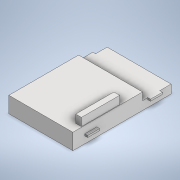
# Autodesk Inventor part: Screen_Model
Saved by Autodesk Inventor 2021 (Build 250183000, 183)
## iProperties
Created: 2020-07-08
Part Number: Screen_Model
Material: Generic
Document SubType Name: Modeling
Designer: ameli
Density: 1 g/cm^3
Appearance: Default
Author: ameli
Autodesk Inventor part; units mm, degrees
ref_plane "YZ Plane" through (0, 0, 0) normal (1, 0, 0) x (0, 1, 0)
ref_plane "XZ Plane" through (0, 0, 0) normal (0, 1, 0) x (-1, 0, 0)
ref_plane "XY Plane" through (0, 0, 0) normal (0, 0, 1) x (1, 0, 0)
sketch "Sketch1" plane through (0, 0, 0) normal (0, 1, 0) x (-1, 0, 0)
  line L0 (28, 43) -> (-28, 43)
  line L1 (-28, 43) -> (-28, -43)
  line L2 (-28, -43) -> (28, -43)
  line L3 (28, -43) -> (28, 43)
  point P0 (0, 0)
  dimension "d0" = 56
  dimension "d1" = 86
  dimension "d4" = 28
  dimension "d5" = 43
  constraints: 8 end point, 2 parallel, 1 horizontal, 1 perpendicular
  measures "d0" distance of L1.end L2.end
  measures "d1" distance of L2.end L0.start
  measures "d4" distance from line of point (0, 0) L3
  measures "d5" distance from line of point (0, 0) L2
extrude "Extrusion1" add sketch "Sketch1" along normal blind 7.5
sketch "Sketch3" plane through (0, 7.5, 0) normal (0, 1, 0) x (1, 0, 0)
  line L0 (22.5, -35) -> (27.5, -35)
  line L1 (27.5, -35) -> (27.5, -1.5)
  line L2 (27.5, -1.5) -> (22.5, -1.5)
  line L3 (22.5, -1.5) -> (22.5, -35)
  line L4 (-28, -43) -> (28, -43) projected
  line L5 (28, -43) -> (28, 43) projected
  point P0 (0, 0)
  dimension "d6" = 33.5
  dimension "d7" = 5
  dimension "d8" = 8
  dimension "d9" = 0.5
  constraints: 8 end point, 2 parallel, 1 horizontal, 1 perpendicular
  measures "d6" distance of L2.end L0.start
  measures "d7" distance of L1.end L2.end
  measures "d8" distance between parallel lines of L4 L0
  measures "d9" distance between parallel lines of L5 L1
extrude "Extrusion2" add sketch "Sketch3" along normal blind 13.5
sketch "Sketch4" plane through (0, 7.5, 0) normal (0, 1, 0) x (1, 0, 0)
  line L0 (-28, 43) -> (-28, -43) projected
  line L1 (-30.4, -32.5) -> (-28, -32.5)
  line L2 (-28, -32.5) -> (-28, -22)
  line L3 (-28, -22) -> (-30.4, -22)
  line L4 (-30.4, -22) -> (-30.4, -32.5)
  line L5 (-30.4, 22.5) -> (-28, 22.5)
  line L6 (-28, 22.5) -> (-28, 33)
  line L7 (-28, 33) -> (-30.4, 33)
  line L8 (-30.4, 33) -> (-30.4, 22.5)
  line L9 (28, -43) -> (28, 43) projected
  line L10 (28, 22.5) -> (30.4, 22.5)
  line L11 (30.4, 22.5) -> (30.4, 33)
  line L12 (30.4, 33) -> (28, 33)
  line L13 (28, 33) -> (28, 22.5)
  line L14 (28, -32.5) -> (30.4, -32.5)
  line L15 (30.4, -32.5) -> (30.4, -22)
  line L16 (30.4, -22) -> (28, -22)
  line L17 (28, -22) -> (28, -32.5)
  line L18 (-28, -43) -> (28, -43) projected
  line L19 (28, 43) -> (-28, 43) projected
  point P0 (0, 0)
  dimension "d12" = 10.5
  dimension "d13" = 10.5
  dimension "d14" = 10.5
  dimension "d15" = 10
  dimension "d16" = 2.4
  dimension "d17" = 2.4
  constraints: 32 end point, 10 point on line, 8 parallel, 4 horizontal, 4 perpendicular
  measures "d12" distance between parallel lines of L3 L1
  measures "d13" distance between parallel lines of L7 L5
  measures "d14" distance between parallel lines of L18 L1
  measures "d15" distance between parallel lines of L19 L7
  measures "d16" distance between parallel lines of L6 L8
  measures "d17" distance between parallel lines of L15 L9
extrude "Extrusion3" add sketch "Sketch4" against normal blind 1.6 contours L0 L5 L8 L7 | L12 L11 L10 L9 | L0 L1 L4 L3 | L16 L15 L14 L9
sketch "Sketch5" plane through (0, 7.5, 0) normal (0, 1, 0) x (1, 0, 0)
  line L0 (-28, 43) -> (-28, -43) projected
  line L1 (28, -22) -> (28, 22.5) projected
  line L2 (-28, -43) -> (28, -43)
  line L3 (28, -43) -> (28, 18)
  line L4 (28, 18) -> (-28, 18)
  line L5 (-28, 18) -> (-28, -43)
  line L6 (28, 43) -> (-28, 43) projected
  point P0 (0, 0)
  dimension "d20" = 25
  constraints: 8 end point, 2 parallel, 1 perpendicular, 1 point on line
  measures "d20" distance between parallel lines of L6 L4
extrude "Extrusion4" add sketch "Sketch5" along normal blind 6.5
body "Solid1"
